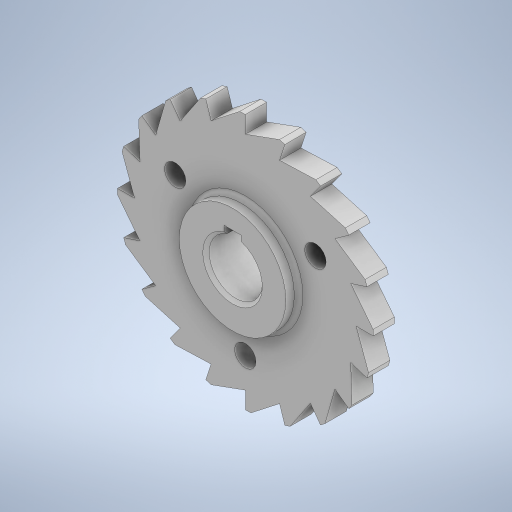
# Autodesk Inventor part: Piesa 35
Saved by Autodesk Inventor 2023 (Build 270158000, 158)
## iProperties
Created: 2023-03-19
Part Number: Piesa 35
Material: Generic
Document SubType Name: Modeling
Designer: Bogdan
Density: 1 g/cm^3
Appearance: Default
Author: Bogdan
Autodesk Inventor part; units mm, degrees
ref_plane "YZ Plane" through (0, 0, 0) normal (1, 0, 0) x (0, 1, 0)
ref_plane "XZ Plane" through (0, 0, 0) normal (0, 1, 0) x (-1, 0, 0)
ref_plane "XY Plane" through (0, 0, 0) normal (0, 0, 1) x (1, 0, 0)
sketch "Sketch1" plane through (0, 0, 0) normal (0, 0, 1) x (1, 0, 0)
  line L0 (-84.0204, 0) -> (84.0204, 0) projected
  line L1 (0, -84.0204) -> (0, 84.0204) projected
  arc A0 (-4, 11.8427) -> (4, 11.8427) centre (0, 0) ccw
  line L2 (0, 16) -> (4, 16)
  line L3 (4, 16) -> (4, 11.8427)
  line L4 (0, 16) -> (-4, 16)
  line L5 (-4, 16) -> (-4, 11.8427)
  circle A1 centre (0, 0) radius 25
  circle A2 centre (0, 0) radius 38 construction
  arc A3 (18.541, 57.0634) -> (16.0059, 57.8257) centre (0, 0) ccw
  circle A4 centre (32.909, 19) radius 5
  line L6 (32.909, 19) -> (0, 0) construction
  circle A5 centre (-32.909, 19) radius 5
  circle A6 centre (0, -38) radius 5
  line L7 (0, 60) -> (0, 52)
  line L8 (0, 52) -> (16.0059, 57.8257)
  line L9 (18.541, 57.0634) -> (16.0689, 49.4549)
  line L10 (-16.0689, 49.4549) -> (-2.6466, 59.9416)
  arc A7 (0, 60) -> (-2.6466, 59.9416) centre (0, 0) ccw
  line L11 (0, 60) -> (0, 52)
  line L12 (-30.5648, 42.0689) -> (-21.04, 56.19)
  arc A8 (-18.541, 57.0634) -> (-21.04, 56.19) centre (0, 0) ccw
  line L13 (-18.541, 57.0634) -> (-16.0689, 49.4549)
  line L14 (-42.0689, 30.5648) -> (-37.3739, 46.9382)
  arc A9 (-35.2671, 48.541) -> (-37.3739, 46.9382) centre (0, 0) ccw
  line L15 (-35.2671, 48.541) -> (-30.5648, 42.0689)
  line L16 (-49.4549, 16.0689) -> (-50.0494, 33.0917)
  arc A10 (-48.541, 35.2671) -> (-50.0494, 33.0917) centre (0, 0) ccw
  line L17 (-48.541, 35.2671) -> (-42.0689, 30.5648)
  line L18 (-52, 0) -> (-57.8257, 16.0059)
  arc A11 (-57.0634, 18.541) -> (-57.8257, 16.0059) centre (0, 0) ccw
  line L19 (-57.0634, 18.541) -> (-49.4549, 16.0689)
  line L20 (-49.4549, -16.0689) -> (-59.9416, -2.6466)
  arc A12 (-60, 0) -> (-59.9416, -2.6466) centre (0, 0) ccw
  line L21 (-60, 0) -> (-52, 0)
  line L22 (-42.0689, -30.5648) -> (-56.19, -21.04)
  arc A13 (-57.0634, -18.541) -> (-56.19, -21.04) centre (0, 0) ccw
  line L23 (-57.0634, -18.541) -> (-49.4549, -16.0689)
  line L24 (-30.5648, -42.0689) -> (-46.9382, -37.3739)
  arc A14 (-48.541, -35.2671) -> (-46.9382, -37.3739) centre (0, 0) ccw
  line L25 (-48.541, -35.2671) -> (-42.0689, -30.5648)
  line L26 (-16.0689, -49.4549) -> (-33.0917, -50.0494)
  arc A15 (-35.2671, -48.541) -> (-33.0917, -50.0494) centre (0, 0) ccw
  line L27 (-35.2671, -48.541) -> (-30.5648, -42.0689)
  line L28 (0, -52) -> (-16.0059, -57.8257)
  arc A16 (-18.541, -57.0634) -> (-16.0059, -57.8257) centre (0, 0) ccw
  line L29 (-18.541, -57.0634) -> (-16.0689, -49.4549)
  line L30 (16.0689, -49.4549) -> (2.6466, -59.9416)
  arc A17 (0, -60) -> (2.6466, -59.9416) centre (0, 0) ccw
  line L31 (0, -60) -> (0, -52)
  line L32 (30.5648, -42.0689) -> (21.04, -56.19)
  arc A18 (18.541, -57.0634) -> (21.04, -56.19) centre (0, 0) ccw
  line L33 (18.541, -57.0634) -> (16.0689, -49.4549)
  line L34 (42.0689, -30.5648) -> (37.3739, -46.9382)
  arc A19 (35.2671, -48.541) -> (37.3739, -46.9382) centre (0, 0) ccw
  line L35 (35.2671, -48.541) -> (30.5648, -42.0689)
  line L36 (49.4549, -16.0689) -> (50.0494, -33.0917)
  arc A20 (48.541, -35.2671) -> (50.0494, -33.0917) centre (0, 0) ccw
  line L37 (48.541, -35.2671) -> (42.0689, -30.5648)
  line L38 (52, 0) -> (57.8257, -16.0059)
  arc A21 (57.0634, -18.541) -> (57.8257, -16.0059) centre (0, 0) ccw
  line L39 (57.0634, -18.541) -> (49.4549, -16.0689)
  line L40 (49.4549, 16.0689) -> (59.9416, 2.6466)
  arc A22 (60, 0) -> (59.9416, 2.6466) centre (0, 0) ccw
  line L41 (60, 0) -> (52, 0)
  line L42 (42.0689, 30.5648) -> (56.19, 21.04)
  arc A23 (57.0634, 18.541) -> (56.19, 21.04) centre (0, 0) ccw
  line L43 (57.0634, 18.541) -> (49.4549, 16.0689)
  line L44 (30.5648, 42.0689) -> (46.9382, 37.3739)
  arc A24 (48.541, 35.2671) -> (46.9382, 37.3739) centre (0, 0) ccw
  line L45 (48.541, 35.2671) -> (42.0689, 30.5648)
  line L46 (16.0689, 49.4549) -> (33.0917, 50.0494)
  arc A25 (35.2671, 48.541) -> (33.0917, 50.0494) centre (0, 0) ccw
  line L47 (35.2671, 48.541) -> (30.5648, 42.0689)
  point P0 (0, -12.5)
  point P1 (-2, 16)
  point P2 (17.305, 53.2592)
  point P3 (0, 56)
  point P4 (-17.305, 53.2592)
  point P5 (-32.916, 45.305)
  point P6 (-45.305, 32.916)
  point P7 (-53.2592, 17.305)
  point P8 (-56, 0)
  point P9 (-53.2592, -17.305)
  point P10 (-45.305, -32.916)
  point P11 (-32.916, -45.305)
  point P12 (-17.305, -53.2592)
  point P13 (0, -56)
  point P14 (17.305, -53.2592)
  point P15 (32.916, -45.305)
  point P16 (45.305, -32.916)
  point P17 (53.2592, -17.305)
  point P18 (56, 0)
  point P19 (53.2592, 17.305)
  point P20 (45.305, 32.916)
  point P21 (32.916, 45.305)
  point P22 (-60, 0)
  point P23 (0, -60)
  point P24 (60, 0)
  dimension "d4" = 76
  dimension "d0" = 25
  dimension "d1" = 8
  dimension "d2" = 28.5
  dimension "d3" = 50
  dimension "d5" = 120
  dimension "d6" = 10
  dimension "d7" = 60
  dimension "d10" = 360
  dimension "d12" = 8
  dimension "d13" = 70
  dimension "d14" = 8
  dimension "d15" = 18
  dimension "d19" = 360
  dimension "d21" = 17.0332
  constraints: 92 end point, 43 point on circle, 25 centre point, 5 point on line, 4 coincident, 3 perpendicular, 2 collinear, 2 midpoint, 191 other
  measures "d0" diameter of A0
  measures "d1" distance of L2.end L4.end
  measures "d2" vertical distance of point (0, -12.5) point (-2, 16)
  measures "d3" diameter of A1
  measures "d5" diameter of A3
  measures "d6" diameter of A4
  measures "d7" angle of L6 L1
  measures "d12" distance of L7.start L7.end
  measures "d13" angle of L8 L7
  measures "d14" distance of L9.start L9.end
  measures "d21" distance of L18.start L18.end
extrude "Extrusion1" add sketch "Sketch1" along normal mid plane 22 contours A1 L1 L4 L5 A0 L0 | L0 A0 L1 A1 | A1 L0 A0 L3 L2 L1 | L1 A0 L0 A1
extrude "Extrusion2" add sketch "Sketch1" along normal mid plane 10 contours L0 A1 L1 A6 L28 A16 L29 L26 A15 L27 L24 A14 L25 L22 A13 L23 L20 A12 | L18 A11 L19 L16 A10 L17 L14 A9 L15 L12 A8 L13 L10 A7 L1 A1 L0 | L1 L8 A3 L9 L46 A25 L47 L44 A24 L45 L42 A23 L43 L40 A22 L0 A1 | A1 L0 L38 A21 L39 L36 A20 L37 L34 A19 L35 L32 A18 L33 L30 A17 L1 A6
fillet "Fillet1" radius 2 2 edges at (-25, 0, 5) (-25, 0, -5)
chamfer "Chamfer1" distance 1.5 angle 45 2 edges at (0, -12.5, 11) (0, -12.5, -11) measured on face at (-4.9522, 11.4772, 3.6667)
body "Solid1"
